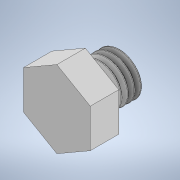
# Autodesk Inventor part: 2020-5_8x11ExternalBolt1A
Saved by Autodesk Inventor 2021.1 (Build 251245010, 245A)
## iProperties
Created: 2020-10-19
Part Number: 2020-5_8x11ExternalBolt1A
Material: Generic
Document SubType Name: Modeling
Designer: robst
Density: 1 g/cm^3
Appearance: Default
Author: robst
Autodesk Inventor part; units mm, degrees
ref_plane "YZ Plane" through (0, 0, 0) normal (1, 0, 0) x (0, 1, 0)
ref_plane "XZ Plane" through (0, 0, 0) normal (0, 1, 0) x (-1, 0, 0)
ref_plane "XY Plane" through (0, 0, 0) normal (0, 0, 1) x (1, 0, 0)
sketch "Sketch1" plane through (0, 0, 0) normal (0, 0, 1) x (1, 0, 0)
  line L0 (11.9062, 6.8741) -> (11.9062, -6.8741)
  line L1 (11.9062, -6.8741) -> (0, -13.7482)
  line L2 (0, -13.7482) -> (-11.9062, -6.8741)
  line L3 (-11.9062, -6.8741) -> (-11.9063, 6.8741)
  line L4 (-11.9063, 6.8741) -> (0, 13.7482)
  line L5 (0, 13.7482) -> (11.9062, 6.8741)
  point P0 (0, 0)
  point P1 (0, 0)
  dimension "d0" = 23.8125
  constraints: 12 end point, 1 coincident, 1 vertical, 13 other
  measures "d0" distance between parallel lines of L3 L0
extrude "Extrusion1" add sketch "Sketch1" along normal blind 10.16
sketch "Sketch2" plane through (0, 0, 0) normal (0, 0, -1) x (-1, 0, 0)
  circle A0 centre (0, 0) radius 7.8016
  dimension "d3" = 15.6032
  constraints: 1 centre point, 1 coincident
  measures "d3" diameter of A0
extrude "Extrusion2" add sketch "Sketch2" along normal blind 12.7
thread "Thread1" size "5/8-11 UNC" class "1A" standard "ANSI Unified Screw Threads" full length
sketch "Sketch4" plane through (0, 0, -12.7) normal (1, 0, 0) x (0, 1, 0)
  line L0 (7.8016, 0) -> (7.8016, 12.7)
  line L1 (7.8016, 12.7) -> (6.0895, 12.7)
  line L2 (6.0895, 12.7) -> (6.0895, 0)
  line L3 (6.0895, 0) -> (7.8016, 0)
  line L4 (0, -7.5935) -> (0, 27.9356) projected
  constraints: 8 end point
revolve "Revolution1" cut sketch "Sketch4" angle 360 about axis through (0, 0, -12.7) along (0, 0, 1)
sketch "Sketch5" plane through (0, 0, -12.7) normal (1, 0, 0) x (0, 1, 0)
  line L0 (7.8016, 0) -> (7.8016, 12.7)
  line L1 (7.8016, 12.7) -> (6.0895, 12.7)
  line L2 (6.0895, 12.7) -> (6.0895, 0)
  line L3 (6.0895, 0) -> (7.8016, 0)
  line L4 (0, -7.5935) -> (0, 27.9356) projected
  constraints: 8 end point
revolve "Revolution2" add sketch "Sketch5" angle 360 about axis through (0, 0, -12.7) along (0, 0, 1) separate body
sketch "Sketch3" plane through (0, 0, -12.7) normal (-1, 0, 0) x (0, 0, 1)
  line L0 (-1.3471, -6.2064) -> (-1.1546, -6.2064) construction
  line L1 (0.1923, -7.685) -> (-0.0001, -8.0547) construction
  line L2 (-2.3092, -8.0547) -> (-2.5016, -7.685) construction
  line L3 (-0.9622, -6.2064) -> (-1.1546, -5.8368) construction
  line L4 (-1.1546, -5.8368) -> (-1.3471, -6.2064) construction
  line L5 (-2.3092, -8.0547) -> (-2.1168, -7.685) construction
  line L6 (-0.9622, -6.2064) -> (-0.1925, -7.685)
  line L7 (-2.5016, -7.685) -> (-2.1168, -7.685) construction
  arc A0 (-2.5016, -7.685) -> (-2.3092, -7.8018) centre (-2.3092, -7.5848) ccw construction
  line L8 (0.1923, -7.685) -> (-0.1925, -7.685) construction
  line L9 (-2.3092, -8.0547) -> (-2.3092, -7.685) construction
  line L10 (-0.0001, -8.0547) -> (-0.0001, -7.685) construction
  line L11 (-1.1546, -5.8368) -> (-1.1546, -6.0897) construction
  line L12 (-2.3092, -7.8018) -> (-0.0001, -7.8018)
  arc A1 (-2.3092, -7.8018) -> (-2.1168, -7.685) centre (-2.3092, -7.5848) ccw
  line L13 (-0.1925, -7.685) -> (-0.0001, -8.0547) construction
  line L14 (-2.1168, -7.685) -> (-1.3471, -6.2064)
  line L15 (-0.0001, -0.0002) -> (-0.0001, 0.0177)
  line L16 (-0.0001, 0.0177) -> (-0.0001, -0.0002)
  line L17 (-0.0001, -0.0002) -> (0.0334, -0.0002)
  arc A2 (-0.1925, -7.685) -> (-0.0001, -7.8018) centre (-0.0001, -7.5848) ccw
  arc A3 (-0.0001, -7.8018) -> (0.1923, -7.685) centre (-0.0001, -7.5848) ccw construction
  arc A4 (-1.1546, -6.0897) -> (-1.3471, -6.2064) centre (-1.1546, -6.3066) ccw
  arc A5 (-0.9622, -6.2064) -> (-1.1546, -6.0897) centre (-1.1546, -6.3066) ccw
  line L18 (-1.1546, -6.0897) -> (-1.1546, -6.2064) construction
  line L19 (-1.1546, -6.2064) -> (-0.9622, -6.2064) construction
  dimension "d8" = 55
  dimension "d9" = 0.3696
  dimension "d10" = 0.3696
  dimension "Sketch3_ThreadOffset" = 0
  dimension "Sketch3_MajorRadius" = 7.8016
  dimension "d13" = 2.3091
  dimension "Sketch3_MinorRadius" = 6.0895
  constraints: 40 end point, 12 point on circle, 10 parallel, 8 tangent, 6 centre point, 6 collinear, 2 midpoint, 2 point on line, 1 horizontal, 1 perpendicular, 3 other
  measures "d8" angle of L6 L14
  measures "d9" distance of L3.end L0.end
  measures "d10" distance of L1.end L10.end
  measures "Sketch3_ThreadOffset" distance between parallel lines of L15 L10
  measures "Sketch3_MajorRadius" distance from line of L12 L15.start
  measures "d13" distance from line of L1.end L9
  measures "Sketch3_MinorRadius" distance edge to line of A5 L17
coil "Coil1" sketch "Sketch3" operation cut axis through (0, 0, -12.7) along (0, 0, 1) pitch 2.3114 turns 7.492507 hand right bodies 2
equation "\"d8\" = d15"
equation "\"d9\" = 0.160083 * Sketch3_Pitch"
equation "\"d10\" = 0.160083 * Sketch3_Pitch"
equation "\"d13\" = Sketch3_Pitch"
equation "\"d15\" = 55deg"
equation "\"Sketch3_Pitch\" = 2.30909"
body "Solid1"
body "Solid2"
